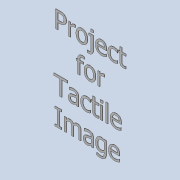
# Autodesk Inventor part: Tactile image
Saved by Autodesk Inventor 2020 (Build 240168000, 168)
## iProperties
Created: 2021-01-22
Part Number: Tactile image
Material: Generic
Document SubType Name: Modeling
Designer: Iulian Bors
Density: 1 g/cm^3
Appearance: Default
Author: Iulian Bors
Autodesk Inventor part; units mm, degrees
ref_plane "YZ Plane" through (0, 0, 0) normal (1, 0, 0) x (0, 1, 0)
ref_plane "XZ Plane" through (0, 0, 0) normal (0, 1, 0) x (-1, 0, 0)
ref_plane "XY Plane" through (0, 0, 0) normal (0, 0, 1) x (1, 0, 0)
sketch "Sketch1" plane through (0, 0, 0) normal (0, 0, 1) x (1, 0, 0)
  line L0 (-100, 150) -> (100, 150)
  line L1 (100, 150) -> (100, -150)
  line L2 (100, -150) -> (-100, -150)
  line L3 (-100, -150) -> (-100, 150)
  line L4 (-57.8261, 112.377) -> (-43.9026, 112.377) construction
  line L5 (-43.9026, 112.377) -> (-43.9026, 98.4276) construction
  line L6 (-43.9026, 98.4276) -> (-57.8261, 98.4276) construction
  line L7 (-57.8261, 98.4276) -> (-57.8261, 112.377) construction
  line L8 (-25, -80) -> (25, -80)
  line L9 (25, -80) -> (25, -130)
  line L10 (25, -130) -> (-25, -130)
  line L11 (-25, -130) -> (-25, -80)
  spline S0 degree 2 poles (-39.4914, 104.6785) (-39.4914, 103.0577) (-40.6462, 100.1404) (-41.6794, 99.1274) knots 0 0 0 1 2 2 2
  spline S1 degree 2 poles (-41.6794, 99.1274) (-42.976, 97.8511) (-46.4809, 96.5342) (-49.1551, 96.5342) knots 0 0 0 1 2 2 2
  line L12 (-49.1551, 96.5342) -> (-51.9711, 96.5342)
  line L13 (-51.9711, 96.5342) -> (-51.9711, 87.2149)
  line L14 (-51.9711, 87.2149) -> (-55.2937, 87.2149)
  line L15 (-55.2937, 87.2149) -> (-55.2937, 112.2149)
  line L16 (-55.2937, 112.2149) -> (-49.0133, 112.2149)
  spline S2 degree 2 poles (-49.0133, 112.2149) (-46.7848, 112.2149) (-43.6648, 111.4856) (-42.4695, 110.655) knots 0 0 0 1 2 2 2
  spline S3 degree 2 poles (-42.4695, 110.655) (-41.0716, 109.7028) (-39.4914, 106.7652) (-39.4914, 104.6785) knots 0 0 0 1 2 2 2
  spline S4 degree 2 poles (-42.9557, 104.5772) (-42.9557, 105.8738) (-43.8472, 107.7781) (-44.7588, 108.3859) knots 0 0 0 1 2 2 2
  spline S5 degree 2 poles (-44.7588, 108.3859) (-45.5489, 108.9127) (-47.6559, 109.3381) (-49.2159, 109.3381) knots 0 0 0 1 2 2 2
  line L17 (-49.2159, 109.3381) -> (-51.9711, 109.3381)
  line L18 (-51.9711, 109.3381) -> (-51.9711, 99.3705)
  line L19 (-51.9711, 99.3705) -> (-49.7021, 99.3705)
  spline S6 degree 2 poles (-49.7021, 99.3705) (-47.6762, 99.3705) (-45.1843, 100.0188) (-44.3739, 100.8697) knots 0 0 0 1 2 2 2
  spline S7 degree 2 poles (-44.3739, 100.8697) (-43.6243, 101.6193) (-42.9557, 103.3819) (-42.9557, 104.5772) knots 0 0 0 1 2 2 2
  line L20 (-26.6267, 102.5918) -> (-26.7888, 102.5918)
  spline S8 degree 2 poles (-26.7888, 102.5918) (-27.1535, 102.6931) (-27.9436, 102.7336) (-28.4906, 102.7336) knots 0 0 0 1 2 2 2
  spline S9 degree 2 poles (-28.4906, 102.7336) (-29.7669, 102.7336) (-32.2791, 101.6193) (-33.4136, 100.5253) knots 0 0 0 1 2 2 2
  line L21 (-33.4136, 100.5253) -> (-33.4136, 87.2149)
  line L22 (-33.4136, 87.2149) -> (-36.5741, 87.2149)
  line L23 (-36.5741, 87.2149) -> (-36.5741, 105.9751)
  line L24 (-36.5741, 105.9751) -> (-33.4136, 105.9751)
  line L25 (-33.4136, 105.9751) -> (-33.4136, 103.1793)
  spline S10 degree 2 poles (-33.4136, 103.1793) (-31.6916, 104.719) (-29.1186, 105.9751) (-27.9031, 105.9751) knots 0 0 0 1 2 2 2
  spline S11 degree 2 poles (-27.9031, 105.9751) (-27.4168, 105.9751) (-26.9306, 105.9345) (-26.6267, 105.8738) knots 0 0 0 1 2 2 2
  line L26 (-26.6267, 105.8738) -> (-26.6267, 102.5918)
  spline S12 degree 2 poles (-8.758, 96.595) (-8.758, 91.8543) (-13.3164, 86.6882) (-17.1251, 86.6882) knots 0 0 0 1 2 2 2
  spline S13 degree 2 poles (-17.1251, 86.6882) (-21.0352, 86.6882) (-25.5125, 92.0164) (-25.5125, 96.595) knots 0 0 0 1 2 2 2
  spline S14 degree 2 poles (-25.5125, 96.595) (-25.5125, 101.2952) (-20.8933, 106.5018) (-17.1251, 106.5018) knots 0 0 0 1 2 2 2
  spline S15 degree 2 poles (-17.1251, 106.5018) (-13.3164, 106.5018) (-8.758, 101.3154) (-8.758, 96.595) knots 0 0 0 1 2 2 2
  spline S16 degree 2 poles (-12.0198, 96.595) (-12.0198, 100.2417) (-14.6737, 103.7871) (-17.1251, 103.7871) knots 0 0 0 1 2 2 2
  spline S17 degree 2 poles (-17.1251, 103.7871) (-19.5765, 103.7871) (-22.2507, 100.2417) (-22.2507, 96.595) knots 0 0 0 1 2 2 2
  spline S18 degree 2 poles (-22.2507, 96.595) (-22.2507, 93.0496) (-19.5765, 89.4029) (-17.1251, 89.4029) knots 0 0 0 1 2 2 2
  spline S19 degree 2 poles (-17.1251, 89.4029) (-14.694, 89.4029) (-12.0198, 92.9888) (-12.0198, 96.595) knots 0 0 0 1 2 2 2
  spline S20 degree 2 poles (-0.4112, 86.6882) (-0.4112, 83.4872) (-3.8553, 80.1242) (-6.8739, 80.1242) knots 0 0 0 1 2 2 2
  spline S21 degree 2 poles (-6.8739, 80.1242) (-7.4006, 80.1242) (-8.6972, 80.2255) (-9.3253, 80.3268) knots 0 0 0 1 2 2 2
  line L27 (-9.3253, 80.3268) -> (-9.3253, 83.1631)
  line L28 (-9.3253, 83.1631) -> (-9.1429, 83.1631)
  spline S22 degree 2 poles (-9.1429, 83.1631) (-8.7783, 83.082) (-7.8869, 82.92) (-7.4817, 82.92) knots 0 0 0 1 2 2 2
  spline S23 degree 2 poles (-7.4817, 82.92) (-6.2256, 82.92) (-4.5846, 83.548) (-4.1997, 84.2166) knots 0 0 0 1 2 2 2
  spline S24 degree 2 poles (-4.1997, 84.2166) (-3.8147, 84.8243) (-3.5716, 86.6679) (-3.5716, 87.9848) knots 0 0 0 1 2 2 2
  line L29 (-3.5716, 87.9848) -> (-3.5716, 103.3616)
  line L30 (-3.5716, 103.3616) -> (-6.9549, 103.3616)
  line L31 (-6.9549, 103.3616) -> (-6.9549, 105.9751)
  line L32 (-6.9549, 105.9751) -> (-0.4112, 105.9751)
  line L33 (-0.4112, 105.9751) -> (-0.4112, 86.6882)
  line L34 (-0.3909, 109.095) -> (-3.9768, 109.095)
  line L35 (-3.9768, 109.095) -> (-3.9768, 112.377)
  line L36 (-3.9768, 112.377) -> (-0.3909, 112.377)
  line L37 (-0.3909, 112.377) -> (-0.3909, 109.095)
  spline S25 degree 2 poles (12.3117, 86.7895) (7.8141, 86.7895) (2.8708, 91.8341) (2.8708, 96.4937) knots 0 0 0 1 2 2 2
  spline S26 degree 2 poles (2.8708, 96.4937) (2.8708, 101.0723) (7.6723, 106.5018) (11.5418, 106.5018) knots 0 0 0 1 2 2 2
  spline S27 degree 2 poles (11.5418, 106.5018) (13.2841, 106.5018) (15.9786, 105.4888) (16.9713, 104.4151) knots 0 0 0 1 2 2 2
  spline S28 degree 2 poles (16.9713, 104.4151) (17.9843, 103.3413) (19.058, 100.2417) (19.058, 97.9929) knots 0 0 0 1 2 2 2
  line L38 (19.058, 97.9929) -> (19.058, 96.2708)
  line L39 (19.058, 96.2708) -> (6.0718, 96.2708)
  spline S29 degree 2 poles (6.0718, 96.2708) (6.0718, 93.0091) (9.3538, 89.5448) (12.2712, 89.5448) knots 0 0 0 1 2 2 2
  spline S30 degree 2 poles (12.2712, 89.5448) (13.3044, 89.5448) (15.3101, 90.0107) (16.1204, 90.3754) knots 0 0 0 1 2 2 2
  spline S31 degree 2 poles (16.1204, 90.3754) (16.9713, 90.7806) (18.1464, 91.4896) (18.5313, 91.8138) knots 0 0 0 1 2 2 2
  line L40 (18.5313, 91.8138) -> (18.7136, 91.8138)
  line L41 (18.7136, 91.8138) -> (18.7136, 88.3697)
  spline S32 degree 2 poles (18.7136, 88.3697) (18.1666, 88.1469) (16.5054, 87.4986) (15.8571, 87.3162) knots 0 0 0 1 2 2 2
  spline S33 degree 2 poles (15.8571, 87.3162) (14.9454, 87.0529) (13.4462, 86.7895) (12.3117, 86.7895) knots 0 0 0 1 2 2 2
  spline S34 degree 2 poles (15.9786, 98.6817) (15.9381, 99.958) (15.4114, 101.8219) (14.9049, 102.4499) knots 0 0 0 1 2 2 2
  spline S35 degree 2 poles (14.9049, 102.4499) (14.3579, 103.159) (12.6358, 103.9086) (11.3595, 103.9086) knots 0 0 0 1 2 2 2
  spline S36 degree 2 poles (11.3595, 103.9086) (10.1034, 103.9086) (8.3408, 103.159) (7.6115, 102.4297) knots 0 0 0 1 2 2 2
  spline S37 degree 2 poles (7.6115, 102.4297) (6.9024, 101.6801) (6.1731, 99.877) (6.0718, 98.6817) knots 0 0 0 1 2 2 2
  line L42 (6.0718, 98.6817) -> (15.9786, 98.6817)
  spline S38 degree 2 poles (29.7144, 86.7895) (27.7695, 86.7895) (24.5483, 87.9848) (23.3935, 89.2003) knots 0 0 0 1 2 2 2
  spline S39 degree 2 poles (23.3935, 89.2003) (22.2387, 90.3956) (20.9624, 94.0828) (20.9624, 96.5545) knots 0 0 0 1 2 2 2
  spline S40 degree 2 poles (20.9624, 96.5545) (20.9624, 99.0261) (22.2793, 102.6323) (23.3935, 103.8478) knots 0 0 0 1 2 2 2
  spline S41 degree 2 poles (23.3935, 103.8478) (24.5078, 105.0837) (27.8101, 106.4005) (29.7144, 106.4005) knots 0 0 0 1 2 2 2
  spline S42 degree 2 poles (29.7144, 106.4005) (31.2541, 106.4005) (34.131, 105.5294) (35.2452, 104.9621) knots 0 0 0 1 2 2 2
  line L43 (35.2452, 104.9621) -> (35.2452, 101.4167)
  line L44 (35.2452, 101.4167) -> (35.0629, 101.4167)
  spline S43 degree 2 poles (35.0629, 101.4167) (34.7185, 101.7003) (33.665, 102.4297) (32.9154, 102.8146) knots 0 0 0 1 2 2 2
  spline S44 degree 2 poles (32.9154, 102.8146) (32.2468, 103.1388) (30.464, 103.6452) (29.6537, 103.6452) knots 0 0 0 1 2 2 2
  spline S45 degree 2 poles (29.6537, 103.6452) (27.2023, 103.6452) (24.2242, 99.9378) (24.2242, 96.5545) knots 0 0 0 1 2 2 2
  spline S46 degree 2 poles (24.2242, 96.5545) (24.2242, 93.2522) (27.101, 89.5448) (29.6537, 89.5448) knots 0 0 0 1 2 2 2
  spline S47 degree 2 poles (29.6537, 89.5448) (31.1934, 89.5448) (33.9891, 90.8211) (35.0629, 91.8138) knots 0 0 0 1 2 2 2
  line L45 (35.0629, 91.8138) -> (35.2452, 91.8138)
  line L46 (35.2452, 91.8138) -> (35.2452, 88.2684)
  spline S48 degree 2 poles (35.2452, 88.2684) (34.7793, 88.0456) (33.3611, 87.4175) (32.7938, 87.2757) knots 0 0 0 1 2 2 2
  spline S49 degree 2 poles (32.7938, 87.2757) (31.9835, 87.0326) (30.7071, 86.7895) (29.7144, 86.7895) knots 0 0 0 1 2 2 2
  spline S50 degree 2 poles (43.7947, 86.8503) (41.2217, 86.8503) (38.3246, 89.7879) (38.3246, 92.9686) knots 0 0 0 1 2 2 2
  line L47 (38.3246, 92.9686) -> (38.3246, 103.3616)
  line L48 (38.3246, 103.3616) -> (36.1974, 103.3616)
  line L49 (36.1974, 103.3616) -> (36.1974, 105.9751)
  line L50 (36.1974, 105.9751) -> (38.3246, 105.9751)
  line L51 (38.3246, 105.9751) -> (38.3246, 111.364)
  line L52 (38.3246, 111.364) -> (41.4851, 111.364)
  line L53 (41.4851, 111.364) -> (41.4851, 105.9751)
  line L54 (41.4851, 105.9751) -> (47.2995, 105.9751)
  line L55 (47.2995, 105.9751) -> (47.2995, 103.3616)
  line L56 (47.2995, 103.3616) -> (41.4851, 103.3616)
  line L57 (41.4851, 103.3616) -> (41.4851, 94.4272)
  spline S51 degree 2 poles (41.4851, 94.4272) (41.4851, 93.0091) (41.5864, 91.4491) (41.9308, 90.7806) knots 0 0 0 1 2 2 2
  spline S52 degree 2 poles (41.9308, 90.7806) (42.2144, 90.1931) (43.4908, 89.6055) (44.5848, 89.6055) knots 0 0 0 1 2 2 2
  spline S53 degree 2 poles (44.5848, 89.6055) (45.3546, 89.6055) (46.793, 90.0715) (47.1172, 90.2133) knots 0 0 0 1 2 2 2
  line L58 (47.1172, 90.2133) -> (47.2995, 90.2133)
  line L59 (47.2995, 90.2133) -> (47.2995, 87.377)
  spline S54 degree 2 poles (47.2995, 87.377) (46.4081, 87.1339) (44.5848, 86.8503) (43.7947, 86.8503) knots 0 0 0 1 2 2 2
  line L60 (-13.4582, 69.1285) -> (-13.6203, 69.1285)
  spline S55 degree 2 poles (-13.6203, 69.1285) (-14.0457, 69.2905) (-15.6259, 69.5742) (-16.254, 69.5742) knots 0 0 0 1 2 2 2
  spline S56 degree 2 poles (-16.254, 69.5742) (-18.2394, 69.5742) (-19.9412, 67.7913) (-19.9412, 65.4413) knots 0 0 0 1 2 2 2
  line L61 (-19.9412, 65.4413) -> (-19.9412, 64.8132)
  line L62 (-19.9412, 64.8132) -> (-14.7143, 64.8132)
  line L63 (-14.7143, 64.8132) -> (-14.7143, 62.1998)
  line L64 (-14.7143, 62.1998) -> (-19.8399, 62.1998)
  line L65 (-19.8399, 62.1998) -> (-19.8399, 46.0531)
  line L66 (-19.8399, 46.0531) -> (-23.0003, 46.0531)
  line L67 (-23.0003, 46.0531) -> (-23.0003, 62.1998)
  line L68 (-23.0003, 62.1998) -> (-25.1275, 62.1998)
  line L69 (-25.1275, 62.1998) -> (-25.1275, 64.8132)
  line L70 (-25.1275, 64.8132) -> (-23.0003, 64.8132)
  line L71 (-23.0003, 64.8132) -> (-23.0003, 65.4413)
  spline S57 degree 2 poles (-23.0003, 65.4413) (-23.0003, 68.8043) (-19.7386, 72.3294) (-16.6997, 72.3294) knots 0 0 0 1 2 2 2
  spline S58 degree 2 poles (-16.6997, 72.3294) (-15.8285, 72.3294) (-14.147, 72.1471) (-13.4582, 72.0255) knots 0 0 0 1 2 2 2
  line L72 (-13.4582, 72.0255) -> (-13.4582, 69.1285)
  spline S59 degree 2 poles (3.0329, 55.4332) (3.0329, 50.6925) (-1.5254, 45.5263) (-5.3342, 45.5263) knots 0 0 0 1 2 2 2
  spline S60 degree 2 poles (-5.3342, 45.5263) (-9.2442, 45.5263) (-13.7215, 50.8545) (-13.7215, 55.4332) knots 0 0 0 1 2 2 2
  spline S61 degree 2 poles (-13.7215, 55.4332) (-13.7215, 60.1333) (-9.1024, 65.34) (-5.3342, 65.34) knots 0 0 0 1 2 2 2
  spline S62 degree 2 poles (-5.3342, 65.34) (-1.5254, 65.34) (3.0329, 60.1536) (3.0329, 55.4332) knots 0 0 0 1 2 2 2
  spline S63 degree 2 poles (-0.2288, 55.4332) (-0.2288, 59.0798) (-2.8828, 62.6252) (-5.3342, 62.6252) knots 0 0 0 1 2 2 2
  spline S64 degree 2 poles (-5.3342, 62.6252) (-7.7856, 62.6252) (-10.4598, 59.0798) (-10.4598, 55.4332) knots 0 0 0 1 2 2 2
  spline S65 degree 2 poles (-10.4598, 55.4332) (-10.4598, 51.8878) (-7.7856, 48.2411) (-5.3342, 48.2411) knots 0 0 0 1 2 2 2
  spline S66 degree 2 poles (-5.3342, 48.2411) (-2.9031, 48.2411) (-0.2288, 51.827) (-0.2288, 55.4332) knots 0 0 0 1 2 2 2
  line L73 (16.2217, 61.4299) -> (16.0596, 61.4299)
  spline S67 degree 2 poles (16.0596, 61.4299) (15.695, 61.5312) (14.9049, 61.5717) (14.3579, 61.5717) knots 0 0 0 1 2 2 2
  spline S68 degree 2 poles (14.3579, 61.5717) (13.0815, 61.5717) (10.5694, 60.4575) (9.4349, 59.3635) knots 0 0 0 1 2 2 2
  line L74 (9.4349, 59.3635) -> (9.4349, 46.0531)
  line L75 (9.4349, 46.0531) -> (6.2744, 46.0531)
  line L76 (6.2744, 46.0531) -> (6.2744, 64.8132)
  line L77 (6.2744, 64.8132) -> (9.4349, 64.8132)
  line L78 (9.4349, 64.8132) -> (9.4349, 62.0174)
  spline S69 degree 2 poles (9.4349, 62.0174) (11.1569, 63.5571) (13.7298, 64.8132) (14.9454, 64.8132) knots 0 0 0 1 2 2 2
  spline S70 degree 2 poles (14.9454, 64.8132) (15.4316, 64.8132) (15.9178, 64.7727) (16.2217, 64.7119) knots 0 0 0 1 2 2 2
  line L79 (16.2217, 64.7119) -> (16.2217, 61.4299)
  line L80 (-49.459, 4.8912) -> (-49.459, 26.9334)
  line L81 (-49.459, 26.9334) -> (-57.8463, 26.9334)
  line L82 (-57.8463, 26.9334) -> (-57.8463, 29.8912)
  line L83 (-57.8463, 29.8912) -> (-37.7491, 29.8912)
  line L84 (-37.7491, 29.8912) -> (-37.7491, 26.9334)
  line L85 (-37.7491, 26.9334) -> (-46.1365, 26.9334)
  line L86 (-46.1365, 26.9334) -> (-46.1365, 4.8912)
  line L87 (-46.1365, 4.8912) -> (-49.459, 4.8912)
  spline S71 degree 2 poles (-25.006, 6.8767) (-25.3909, 6.593) (-26.6875, 5.5801) (-27.2953, 5.2762) knots 0 0 0 1 2 2 2
  spline S72 degree 2 poles (-27.2953, 5.2762) (-28.1259, 4.8305) (-29.6859, 4.3645) (-31.104, 4.3645) knots 0 0 0 1 2 2 2
  spline S73 degree 2 poles (-31.104, 4.3645) (-32.2588, 4.3645) (-34.3455, 5.2357) (-35.1357, 6.0258) knots 0 0 0 1 2 2 2
  spline S74 degree 2 poles (-35.1357, 6.0258) (-35.8852, 6.7956) (-36.7969, 9.0647) (-36.7969, 10.3207) knots 0 0 0 1 2 2 2
  spline S75 degree 2 poles (-36.7969, 10.3207) (-36.7969, 12.2656) (-35.1559, 15.0209) (-33.3731, 15.811) knots 0 0 0 1 2 2 2
  spline S76 degree 2 poles (-33.3731, 15.811) (-31.7929, 16.5404) (-27.4979, 17.0874) (-25.006, 17.2292) knots 0 0 0 1 2 2 2
  line L88 (-25.006, 17.2292) -> (-25.006, 17.837)
  spline S77 degree 2 poles (-25.006, 17.837) (-25.006, 18.931) (-25.6745, 20.2883) (-26.2823, 20.6733) knots 0 0 0 1 2 2 2
  spline S78 degree 2 poles (-26.2823, 20.6733) (-26.8901, 21.0582) (-28.6324, 21.3013) (-29.5643, 21.3013) knots 0 0 0 1 2 2 2
  spline S79 degree 2 poles (-29.5643, 21.3013) (-30.6583, 21.3013) (-33.6162, 20.653) (-35.0951, 20.025) knots 0 0 0 1 2 2 2
  line L89 (-35.0951, 20.025) -> (-35.2775, 20.025)
  line L90 (-35.2775, 20.025) -> (-35.2775, 23.2462)
  spline S80 degree 2 poles (-35.2775, 23.2462) (-34.4063, 23.4893) (-31.1446, 24.0971) (-29.5441, 24.0971) knots 0 0 0 1 2 2 2
  spline S81 degree 2 poles (-29.5441, 24.0971) (-27.5992, 24.0971) (-24.9452, 23.4893) (-23.8917, 22.6992) knots 0 0 0 1 2 2 2
  spline S82 degree 2 poles (-23.8917, 22.6992) (-22.8585, 21.9293) (-21.8455, 19.478) (-21.8455, 17.7154) knots 0 0 0 1 2 2 2
  line L91 (-21.8455, 17.7154) -> (-21.8455, 4.8912)
  line L92 (-21.8455, 4.8912) -> (-25.006, 4.8912)
  line L93 (-25.006, 4.8912) -> (-25.006, 6.8767)
  line L94 (-25.006, 9.5104) -> (-25.006, 14.717)
  spline S83 degree 2 poles (-25.006, 14.717) (-26.1405, 14.6157) (-29.5643, 14.2713) (-30.6381, 13.9472) knots 0 0 0 1 2 2 2
  spline S84 degree 2 poles (-30.6381, 13.9472) (-31.8942, 13.5622) (-33.5352, 11.9617) (-33.5352, 10.5436) knots 0 0 0 1 2 2 2
  spline S85 degree 2 poles (-33.5352, 10.5436) (-33.5352, 8.9229) (-31.7118, 7.2818) (-29.9695, 7.2818) knots 0 0 0 1 2 2 2
  spline S86 degree 2 poles (-29.9695, 7.2818) (-28.4906, 7.2818) (-26.0595, 8.5582) (-25.006, 9.5104) knots 0 0 0 1 2 2 2
  spline S87 degree 2 poles (-9.9533, 4.4658) (-11.8982, 4.4658) (-15.1194, 5.6611) (-16.2742, 6.8767) knots 0 0 0 1 2 2 2
  spline S88 degree 2 poles (-16.2742, 6.8767) (-17.429, 8.072) (-18.7053, 11.7592) (-18.7053, 14.2308) knots 0 0 0 1 2 2 2
  spline S89 degree 2 poles (-18.7053, 14.2308) (-18.7053, 16.7024) (-17.3885, 20.3086) (-16.2742, 21.5241) knots 0 0 0 1 2 2 2
  spline S90 degree 2 poles (-16.2742, 21.5241) (-15.16, 22.76) (-11.8577, 24.0768) (-9.9533, 24.0768) knots 0 0 0 1 2 2 2
  spline S91 degree 2 poles (-9.9533, 24.0768) (-8.4136, 24.0768) (-5.5368, 23.2057) (-4.4225, 22.6384) knots 0 0 0 1 2 2 2
  line L95 (-4.4225, 22.6384) -> (-4.4225, 19.093)
  line L96 (-4.4225, 19.093) -> (-4.6049, 19.093)
  spline S92 degree 2 poles (-4.6049, 19.093) (-4.9493, 19.3767) (-6.0027, 20.106) (-6.7523, 20.4909) knots 0 0 0 1 2 2 2
  spline S93 degree 2 poles (-6.7523, 20.4909) (-7.4209, 20.8151) (-9.2037, 21.3216) (-10.0141, 21.3216) knots 0 0 0 1 2 2 2
  spline S94 degree 2 poles (-10.0141, 21.3216) (-12.4655, 21.3216) (-15.4436, 17.6141) (-15.4436, 14.2308) knots 0 0 0 1 2 2 2
  spline S95 degree 2 poles (-15.4436, 14.2308) (-15.4436, 10.9285) (-12.5668, 7.2211) (-10.0141, 7.2211) knots 0 0 0 1 2 2 2
  spline S96 degree 2 poles (-10.0141, 7.2211) (-8.4744, 7.2211) (-5.6786, 8.4974) (-4.6049, 9.4901) knots 0 0 0 1 2 2 2
  line L97 (-4.6049, 9.4901) -> (-4.4225, 9.4901)
  line L98 (-4.4225, 9.4901) -> (-4.4225, 5.9447)
  spline S97 degree 2 poles (-4.4225, 5.9447) (-4.8885, 5.7219) (-6.3066, 5.0938) (-6.8739, 4.952) knots 0 0 0 1 2 2 2
  spline S98 degree 2 poles (-6.8739, 4.952) (-7.6843, 4.7089) (-8.9606, 4.4658) (-9.9533, 4.4658) knots 0 0 0 1 2 2 2
  spline S99 degree 2 poles (4.1269, 4.5266) (1.554, 4.5266) (-1.3431, 7.4642) (-1.3431, 10.6449) knots 0 0 0 1 2 2 2
  line L99 (-1.3431, 10.6449) -> (-1.3431, 21.0379)
  line L100 (-1.3431, 21.0379) -> (-3.4703, 21.0379)
  line L101 (-3.4703, 21.0379) -> (-3.4703, 23.6514)
  line L102 (-3.4703, 23.6514) -> (-1.3431, 23.6514)
  line L103 (-1.3431, 23.6514) -> (-1.3431, 29.0404)
  line L104 (-1.3431, 29.0404) -> (1.8173, 29.0404)
  line L105 (1.8173, 29.0404) -> (1.8173, 23.6514)
  line L106 (1.8173, 23.6514) -> (7.6318, 23.6514)
  line L107 (7.6318, 23.6514) -> (7.6318, 21.0379)
  line L108 (7.6318, 21.0379) -> (1.8173, 21.0379)
  line L109 (1.8173, 21.0379) -> (1.8173, 12.1036)
  spline S100 degree 2 poles (1.8173, 12.1036) (1.8173, 10.6854) (1.9186, 9.1254) (2.2631, 8.4569) knots 0 0 0 1 2 2 2
  spline S101 degree 2 poles (2.2631, 8.4569) (2.5467, 7.8694) (3.823, 7.2818) (4.917, 7.2818) knots 0 0 0 1 2 2 2
  spline S102 degree 2 poles (4.917, 7.2818) (5.6869, 7.2818) (7.1253, 7.7478) (7.4494, 7.8896) knots 0 0 0 1 2 2 2
  line L110 (7.4494, 7.8896) -> (7.6318, 7.8896)
  line L111 (7.6318, 7.8896) -> (7.6318, 5.0533)
  spline S103 degree 2 poles (7.6318, 5.0533) (6.7404, 4.8102) (4.917, 4.5266) (4.1269, 4.5266) knots 0 0 0 1 2 2 2
  line L112 (13.1828, 4.8912) -> (10.0224, 4.8912)
  line L113 (10.0224, 4.8912) -> (10.0224, 23.6514)
  line L114 (10.0224, 23.6514) -> (13.1828, 23.6514)
  line L115 (13.1828, 23.6514) -> (13.1828, 4.8912)
  line L116 (13.4057, 26.7713) -> (9.8198, 26.7713)
  line L117 (9.8198, 26.7713) -> (9.8198, 30.0533)
  line L118 (9.8198, 30.0533) -> (13.4057, 30.0533)
  line L119 (13.4057, 30.0533) -> (13.4057, 26.7713)
  line L120 (21.0434, 4.8912) -> (17.883, 4.8912)
  line L121 (17.883, 4.8912) -> (17.883, 31.0055)
  line L122 (17.883, 31.0055) -> (21.0434, 31.0055)
  line L123 (21.0434, 31.0055) -> (21.0434, 4.8912)
  spline S104 degree 2 poles (33.8271, 4.4658) (29.3295, 4.4658) (24.3862, 9.5104) (24.3862, 14.17) knots 0 0 0 1 2 2 2
  spline S105 degree 2 poles (24.3862, 14.17) (24.3862, 18.7486) (29.1877, 24.1781) (33.0572, 24.1781) knots 0 0 0 1 2 2 2
  spline S106 degree 2 poles (33.0572, 24.1781) (34.7995, 24.1781) (37.494, 23.1652) (38.4867, 22.0914) knots 0 0 0 1 2 2 2
  spline S107 degree 2 poles (38.4867, 22.0914) (39.4997, 21.0177) (40.5734, 17.918) (40.5734, 15.6692) knots 0 0 0 1 2 2 2
  line L124 (40.5734, 15.6692) -> (40.5734, 13.9472)
  line L125 (40.5734, 13.9472) -> (27.5872, 13.9472)
  spline S108 degree 2 poles (27.5872, 13.9472) (27.5872, 10.6854) (30.8692, 7.2211) (33.7866, 7.2211) knots 0 0 0 1 2 2 2
  spline S109 degree 2 poles (33.7866, 7.2211) (34.8198, 7.2211) (36.8255, 7.687) (37.6358, 8.0517) knots 0 0 0 1 2 2 2
  spline S110 degree 2 poles (37.6358, 8.0517) (38.4867, 8.4569) (39.6618, 9.166) (40.0467, 9.4901) knots 0 0 0 1 2 2 2
  line L126 (40.0467, 9.4901) -> (40.229, 9.4901)
  line L127 (40.229, 9.4901) -> (40.229, 6.046)
  spline S111 degree 2 poles (40.229, 6.046) (39.682, 5.8232) (38.0208, 5.1749) (37.3725, 4.9925) knots 0 0 0 1 2 2 2
  spline S112 degree 2 poles (37.3725, 4.9925) (36.4608, 4.7292) (34.9616, 4.4658) (33.8271, 4.4658) knots 0 0 0 1 2 2 2
  spline S113 degree 2 poles (37.494, 16.358) (37.4535, 17.6344) (36.9267, 19.4982) (36.4203, 20.1263) knots 0 0 0 1 2 2 2
  spline S114 degree 2 poles (36.4203, 20.1263) (35.8733, 20.8353) (34.1512, 21.5849) (32.8749, 21.5849) knots 0 0 0 1 2 2 2
  spline S115 degree 2 poles (32.8749, 21.5849) (31.6188, 21.5849) (29.8562, 20.8353) (29.1269, 20.106) knots 0 0 0 1 2 2 2
  spline S116 degree 2 poles (29.1269, 20.106) (28.4178, 19.3564) (27.6885, 17.5533) (27.5872, 16.358) knots 0 0 0 1 2 2 2
  line L128 (27.5872, 16.358) -> (37.494, 16.358)
  line L129 (-46.5822, -36.2706) -> (-56.2661, -36.2706)
  line L130 (-56.2661, -36.2706) -> (-56.2661, -33.7179)
  line L131 (-56.2661, -33.7179) -> (-53.0854, -33.7179)
  line L132 (-53.0854, -33.7179) -> (-53.0854, -13.8233)
  line L133 (-53.0854, -13.8233) -> (-56.2661, -13.8233)
  line L134 (-56.2661, -13.8233) -> (-56.2661, -11.2706)
  line L135 (-56.2661, -11.2706) -> (-46.5822, -11.2706)
  line L136 (-46.5822, -11.2706) -> (-46.5822, -13.8233)
  line L137 (-46.5822, -13.8233) -> (-49.7629, -13.8233)
  line L138 (-49.7629, -13.8233) -> (-49.7629, -33.7179)
  line L139 (-49.7629, -33.7179) -> (-46.5822, -33.7179)
  line L140 (-46.5822, -33.7179) -> (-46.5822, -36.2706)
  line L141 (-21.4404, -36.2706) -> (-21.4404, -25.4116)
  spline S117 degree 2 poles (-21.4404, -25.4116) (-21.4404, -24.115) (-21.6429, -21.9067) (-21.9671, -21.299) knots 0 0 0 1 2 2 2
  spline S118 degree 2 poles (-21.9671, -21.299) (-22.2912, -20.6304) (-23.5271, -19.9821) (-24.6008, -19.9821) knots 0 0 0 1 2 2 2
  spline S119 degree 2 poles (-24.6008, -19.9821) (-25.5733, -19.9821) (-27.8018, -21.1774) (-28.9768, -22.3119) knots 0 0 0 1 2 2 2
  spline S120 degree 2 poles (-28.9768, -22.3119) (-28.9566, -22.5956) (-28.916, -23.3857) (-28.916, -23.9124) knots 0 0 0 1 2 2 2
  line L142 (-28.916, -23.9124) -> (-28.916, -36.2706)
  line L143 (-28.916, -36.2706) -> (-32.0765, -36.2706)
  line L144 (-32.0765, -36.2706) -> (-32.0765, -25.4116)
  spline S121 degree 2 poles (-32.0765, -25.4116) (-32.0765, -24.115) (-32.2791, -21.9067) (-32.6032, -21.299) knots 0 0 0 1 2 2 2
  spline S122 degree 2 poles (-32.6032, -21.299) (-32.9274, -20.6304) (-34.1632, -19.9821) (-35.2369, -19.9821) knots 0 0 0 1 2 2 2
  spline S123 degree 2 poles (-35.2369, -19.9821) (-36.2499, -19.9821) (-38.4987, -21.2584) (-39.5522, -22.2511) knots 0 0 0 1 2 2 2
  line L145 (-39.5522, -22.2511) -> (-39.5522, -36.2706)
  line L146 (-39.5522, -36.2706) -> (-42.7126, -36.2706)
  line L147 (-42.7126, -36.2706) -> (-42.7126, -17.5105)
  line L148 (-42.7126, -17.5105) -> (-39.5522, -17.5105)
  line L149 (-39.5522, -17.5105) -> (-39.5522, -19.5769)
  spline S124 degree 2 poles (-39.5522, -19.5769) (-38.3164, -18.3411) (-35.8852, -16.9837) (-34.4266, -16.9837) knots 0 0 0 1 2 2 2
  spline S125 degree 2 poles (-34.4266, -16.9837) (-32.7653, -16.9837) (-30.1924, -18.5032) (-29.5238, -20.2252) knots 0 0 0 1 2 2 2
  spline S126 degree 2 poles (-29.5238, -20.2252) (-28.0854, -18.6247) (-25.3707, -16.9837) (-23.7904, -16.9837) knots 0 0 0 1 2 2 2
  spline S127 degree 2 poles (-23.7904, -16.9837) (-22.5749, -16.9837) (-20.5895, -17.7333) (-19.8601, -18.5842) knots 0 0 0 1 2 2 2
  spline S128 degree 2 poles (-19.8601, -18.5842) (-19.1105, -19.4351) (-18.2799, -21.9878) (-18.2799, -23.9124) knots 0 0 0 1 2 2 2
  line L150 (-18.2799, -23.9124) -> (-18.2799, -36.2706)
  line L151 (-18.2799, -36.2706) -> (-21.4404, -36.2706)
  spline S129 degree 2 poles (-3.3893, -34.2852) (-3.7742, -34.5688) (-5.0708, -35.5818) (-5.6786, -35.8857) knots 0 0 0 1 2 2 2
  spline S130 degree 2 poles (-5.6786, -35.8857) (-6.5092, -36.3314) (-8.0692, -36.7973) (-9.4874, -36.7973) knots 0 0 0 1 2 2 2
  spline S131 degree 2 poles (-9.4874, -36.7973) (-10.6421, -36.7973) (-12.7288, -35.9262) (-13.519, -35.1361) knots 0 0 0 1 2 2 2
  spline S132 degree 2 poles (-13.519, -35.1361) (-14.2686, -34.3662) (-15.1802, -32.0972) (-15.1802, -30.8411) knots 0 0 0 1 2 2 2
  spline S133 degree 2 poles (-15.1802, -30.8411) (-15.1802, -28.8962) (-13.5392, -26.1409) (-11.7564, -25.3508) knots 0 0 0 1 2 2 2
  spline S134 degree 2 poles (-11.7564, -25.3508) (-10.1762, -24.6215) (-5.8812, -24.0745) (-3.3893, -23.9327) knots 0 0 0 1 2 2 2
  line L152 (-3.3893, -23.9327) -> (-3.3893, -23.3249)
  spline S135 degree 2 poles (-3.3893, -23.3249) (-3.3893, -22.2309) (-4.0579, -20.8735) (-4.6656, -20.4886) knots 0 0 0 1 2 2 2
  spline S136 degree 2 poles (-4.6656, -20.4886) (-5.2734, -20.1037) (-7.0157, -19.8605) (-7.9476, -19.8605) knots 0 0 0 1 2 2 2
  spline S137 degree 2 poles (-7.9476, -19.8605) (-9.0416, -19.8605) (-11.9995, -20.5088) (-13.4784, -21.1369) knots 0 0 0 1 2 2 2
  line L153 (-13.4784, -21.1369) -> (-13.6608, -21.1369)
  line L154 (-13.6608, -21.1369) -> (-13.6608, -17.9157)
  spline S138 degree 2 poles (-13.6608, -17.9157) (-12.7896, -17.6725) (-9.5279, -17.0648) (-7.9274, -17.0648) knots 0 0 0 1 2 2 2
  spline S139 degree 2 poles (-7.9274, -17.0648) (-5.9825, -17.0648) (-3.3285, -17.6725) (-2.275, -18.4627) knots 0 0 0 1 2 2 2
  spline S140 degree 2 poles (-2.275, -18.4627) (-1.2418, -19.2325) (-0.2288, -21.6839) (-0.2288, -23.4464) knots 0 0 0 1 2 2 2
  line L155 (-0.2288, -23.4464) -> (-0.2288, -36.2706)
  line L156 (-0.2288, -36.2706) -> (-3.3893, -36.2706)
  line L157 (-3.3893, -36.2706) -> (-3.3893, -34.2852)
  line L158 (-3.3893, -31.6515) -> (-3.3893, -26.4448)
  spline S141 degree 2 poles (-3.3893, -26.4448) (-4.5238, -26.5461) (-7.9476, -26.8905) (-9.0214, -27.2147) knots 0 0 0 1 2 2 2
  spline S142 degree 2 poles (-9.0214, -27.2147) (-10.2775, -27.5996) (-11.9185, -29.2001) (-11.9185, -30.6182) knots 0 0 0 1 2 2 2
  spline S143 degree 2 poles (-11.9185, -30.6182) (-11.9185, -32.239) (-10.0951, -33.88) (-8.3528, -33.88) knots 0 0 0 1 2 2 2
  spline S144 degree 2 poles (-8.3528, -33.88) (-6.8739, -33.88) (-4.4428, -32.6037) (-3.3893, -31.6515) knots 0 0 0 1 2 2 2
  spline S145 degree 2 poles (4.8765, -39.269) (5.2007, -39.4108) (6.4365, -39.8565) (7.2266, -40.0388) knots 0 0 0 1 2 2 2
  spline S146 degree 2 poles (7.2266, -40.0388) (8.0977, -40.2617) (9.5767, -40.5251) (10.4478, -40.5251) knots 0 0 0 1 2 2 2
  spline S147 degree 2 poles (10.4478, -40.5251) (11.9065, -40.5251) (13.9324, -39.7552) (14.4997, -39.0664) knots 0 0 0 1 2 2 2
  spline S148 degree 2 poles (14.4997, -39.0664) (15.0467, -38.3776) (15.4721, -36.5745) (15.4721, -35.4197) knots 0 0 0 1 2 2 2
  line L159 (15.4721, -35.4197) -> (15.4721, -33.7787)
  spline S149 degree 2 poles (15.4721, -33.7787) (14.1958, -34.893) (11.7444, -35.9464) (9.9008, -35.9464) knots 0 0 0 1 2 2 2
  spline S150 degree 2 poles (9.9008, -35.9464) (6.6998, -35.9464) (2.9114, -31.1855) (2.9114, -26.7082) knots 0 0 0 1 2 2 2
  spline S151 degree 2 poles (2.9114, -26.7082) (2.9114, -24.3784) (4.2282, -20.7722) (5.3222, -19.4959) knots 0 0 0 1 2 2 2
  spline S152 degree 2 poles (5.3222, -19.4959) (6.3757, -18.3006) (9.2728, -16.9837) (10.8125, -16.9837) knots 0 0 0 1 2 2 2
  spline S153 degree 2 poles (10.8125, -16.9837) (12.2712, -16.9837) (14.3984, -17.6725) (15.4721, -18.3006) knots 0 0 0 1 2 2 2
  line L160 (15.4721, -18.3006) -> (15.6545, -17.5105)
  line L161 (15.6545, -17.5105) -> (18.6326, -17.5105)
  line L162 (18.6326, -17.5105) -> (18.6326, -34.1231)
  spline S154 degree 2 poles (18.6326, -34.1231) (18.6326, -38.9043) (14.4794, -43.3614) (10.2047, -43.3614) knots 0 0 0 1 2 2 2
  spline S155 degree 2 poles (10.2047, -43.3614) (8.8271, -43.3614) (5.9502, -42.9157) (4.7144, -42.551) knots 0 0 0 1 2 2 2
  line L163 (4.7144, -42.551) -> (4.7144, -39.269)
  line L164 (4.7144, -39.269) -> (4.8765, -39.269)
  line L165 (15.4721, -31.1855) -> (15.4721, -20.8735)
  spline S156 degree 2 poles (15.4721, -20.8735) (14.2971, -20.3063) (12.3117, -19.82) (11.319, -19.82) knots 0 0 0 1 2 2 2
  spline S157 degree 2 poles (11.319, -19.82) (8.9284, -19.82) (6.1731, -23.3452) (6.1731, -26.6474) knots 0 0 0 1 2 2 2
  spline S158 degree 2 poles (6.1731, -26.6474) (6.1731, -29.7674) (8.2598, -33.0291) (10.6099, -33.0291) knots 0 0 0 1 2 2 2
  spline S159 degree 2 poles (10.6099, -33.0291) (11.8457, -33.0291) (14.4389, -32.0567) (15.4721, -31.1855) knots 0 0 0 1 2 2 2
  spline S160 degree 2 poles (31.3554, -36.696) (26.8579, -36.696) (21.9146, -31.6515) (21.9146, -26.9918) knots 0 0 0 1 2 2 2
  spline S161 degree 2 poles (21.9146, -26.9918) (21.9146, -22.4132) (26.7161, -16.9837) (30.5856, -16.9837) knots 0 0 0 1 2 2 2
  spline S162 degree 2 poles (30.5856, -16.9837) (32.3279, -16.9837) (35.0224, -17.9967) (36.0151, -19.0704) knots 0 0 0 1 2 2 2
  spline S163 degree 2 poles (36.0151, -19.0704) (37.028, -20.1442) (38.1018, -23.2439) (38.1018, -25.4926) knots 0 0 0 1 2 2 2
  line L166 (38.1018, -25.4926) -> (38.1018, -27.2147)
  line L167 (38.1018, -27.2147) -> (25.1156, -27.2147)
  spline S164 degree 2 poles (25.1156, -27.2147) (25.1156, -30.4764) (28.3976, -33.9408) (31.3149, -33.9408) knots 0 0 0 1 2 2 2
  spline S165 degree 2 poles (31.3149, -33.9408) (32.3481, -33.9408) (34.3538, -33.4748) (35.1642, -33.1101) knots 0 0 0 1 2 2 2
  spline S166 degree 2 poles (35.1642, -33.1101) (36.0151, -32.705) (37.1901, -31.9959) (37.575, -31.6717) knots 0 0 0 1 2 2 2
  line L168 (37.575, -31.6717) -> (37.7574, -31.6717)
  line L169 (37.7574, -31.6717) -> (37.7574, -35.1158)
  spline S167 degree 2 poles (37.7574, -35.1158) (37.2104, -35.3387) (35.5491, -35.987) (34.9008, -36.1693) knots 0 0 0 1 2 2 2
  spline S168 degree 2 poles (34.9008, -36.1693) (33.9891, -36.4327) (32.49, -36.696) (31.3554, -36.696) knots 0 0 0 1 2 2 2
  spline S169 degree 2 poles (35.0224, -24.8038) (34.9819, -23.5275) (34.4551, -21.6636) (33.9486, -21.0356) knots 0 0 0 1 2 2 2
  spline S170 degree 2 poles (33.9486, -21.0356) (33.4016, -20.3265) (31.6796, -19.5769) (30.4032, -19.5769) knots 0 0 0 1 2 2 2
  spline S171 degree 2 poles (30.4032, -19.5769) (29.1472, -19.5769) (27.3846, -20.3265) (26.6553, -21.0558) knots 0 0 0 1 2 2 2
  spline S172 degree 2 poles (26.6553, -21.0558) (25.9462, -21.8054) (25.2169, -23.6085) (25.1156, -24.8038) knots 0 0 0 1 2 2 2
  line L170 (25.1156, -24.8038) -> (35.0224, -24.8038)
  point P0 (0, 0)
  point P1 (0, 150)
  point P2 (-100, 0)
  point P3 (0, -130)
  point P4 (0, -150)
  dimension "d0" = 300
  dimension "d1" = 200
  dimension "d4" = 50
  dimension "d5" = 50
  dimension "d6" = 20
  constraints: 16 end point, 4 midpoint, 4 parallel, 2 horizontal, 2 perpendicular, 2 vertical alignment, 1 horizontal alignment, 2 other
  measures "d0" distance of L2.end L0.start
  measures "d1" distance of L1.end L2.end
  measures "d4" distance of L8.start L8.end
  measures "d5" distance of L8.end L9.end
  measures "d6" distance between parallel lines of L2 L10
extrude "Extrusion1" add sketch "Sketch1" along normal blind 0.6 contours S0 S1 L12 L13 L14 L15 L16 S2 S3 | L20 S8 S9 L21 L22 L23 L24 L25 S10 S11 L26 | S12 S13 S14 S15 | S20 S21 L27 L28 S22 S23 S24 L29 L30 L31 L32 L33 | L34 L35 L36 L37 | S25 S26 S27 S28 L38 L39 S29 S30 S31 L40 L41 S32 S33 | S38 S39 S40 S41 S42 L43 L44 S43 S44 S45 S46 S47 L45 L46 S48 S49 | S50 L47 L48 L49 L50 L51 L52 L53 L54 L55 L56 L57 S51 S52 S53 L58 L59 S54 | L60 S55 S56 L61 L62 L63 L64 L65 L66 L67 L68 L69 L70 L71 S57 S58 L72 | S59 S60 S61 S62 | L73 S67 S68 L74 L75 L76 L77 L78 S69 S70 L79 | L80 L81 L82 L83 L84 L85 L86 L87 | S71 S72 S73 S74 S75 S76 L88 S77 S78 S79 L89 L90 S80 S81 S82 L91 L92 L93 | S87 S88 S89 S90 S91 L95 L96 S92 S93 S94 S95 S96 L97 L98 S97 S98 | S99 L99 L100 L101 L102 L103 L104 L105 L106 L107 L108 L109 S100 S101 S102 L110 L111 S103 | L112 L113 L114 L115 | L116 L117 L118 L119 | L120 L121 L122 L123 | S104 S105 S106 S107 L124 L125 S108 S109 S110 L126 L127 S111 S112 | L129 L130 L131 L132 L133 L134 L135 L136 L137 L138 L139 L140 | L141 S117 S118 S119 S120 L142 L143 L144 S121 S122 S123 L145 L146 L147 L148 L149 S124 S125 S126 S127 S128 L150 L151 | S129 S130 S131 S132 S133 S134 L152 S135 S136 S137 L153 L154 S138 S139 S140 L155 L156 L157 | S145 S146 S147 S148 L159 S149 S150 S151 S152 S153 L160 L161 L162 S154 S155 L163 L164 | S160 S161 S162 S163 L166 L167 S164 S165 S166 L168 L169 S167 S168
body "Solid1"
